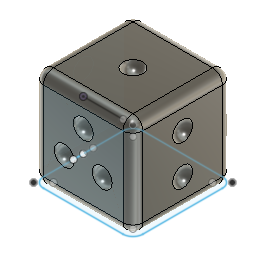
Radial D6 v1 (Autodesk Fusion 360 design; units mm, degrees)
Autodesk Fusion 360 part; units mm, degrees
note: some values were not read from the file. Chosen so that the rebuilt part matches the saved one: which face or edge a step refers to.
sketch "Sketch1" plane through (0, 0, 0) normal (0, 0, 1) x (1, 0, 0)
  line L0 (-20, 25) -> (20, 25)
  line L1 (25, 20) -> (25, -20)
  line L2 (20, -25) -> (-20, -25)
  line L3 (-25, -20) -> (-25, 20)
  arc A0 (-20, 25) -> (-25, 20) centre (-20, 20) ccw
  arc A1 (20, -25) -> (25, -20) centre (20, -20) ccw
  arc A2 (25, 20) -> (20, 25) centre (20, 20) ccw
  arc A3 (-25, -20) -> (-20, -25) centre (-20, -20) ccw
  point P0 (-25, 25)
  point P1 (25, 25)
  point P2 (-25, -25)
  dimension "d1" = 50
  dimension "d2" = 50
  dimension "d3" = 5
  dimension "d4" = 5
  dimension "d5" = 5
  dimension "d6" = 5
  constraint horizontal L0
  constraint vertical L1
  constraint horizontal L2
  constraint vertical L3
  constraint coincident P0 L0
  constraint coincident P0 L3
  constraint tangent L0 A0
  constraint tangent L3 A0
  constraint tangent L1 A1
  constraint tangent L2 A1
  constraint coincident P1 L0
  constraint coincident P1 L1
  constraint tangent L0 A2
  constraint tangent L1 A2
  constraint coincident P2 L2
  constraint coincident P2 L3
  constraint tangent L2 A3
  constraint tangent L3 A3
  measures "d1" distance of P0 P1
  measures "d2" distance of P0 P2
  measures "d3" radius of A0
  measures "d4" radius of A1
  measures "d5" radius of A2
  measures "d6" radius of A3
extrude "Extrude2" add sketch "Sketch1" along normal blind 50
fillet "Fillet3" radius 5 8 edges at (0, 25, 50) (-23.5355, 23.5355, 50) (-25, 0, 50) (-23.5355, -23.5355, 50) (0, -25, 50) (23.5355, -23.5355, 50) (25, 0, 50) (23.5355, 23.5355, 50)
fillet "Fillet4" radius 5 8 edges at (-23.5355, -23.5355, 0) (-25, 0, 0) (-23.5355, 23.5355, 0) (0, 25, 0) (23.5355, 23.5355, 0) (25, 0, 0) (23.5355, -23.5355, 0) (0, -25, 0)
sphere "SpherePrimitive1" cut diameter 10 placed x (-1, 0, 0) y (0, -1, 0) z (0, 0, 1) at (0, 0, 50)
sphere "SpherePrimitive2" cut diameter 10 placed x (1, 0, 0) y (0, 1, 0) z (0, 0, 1) at (13, 0, 0)
pattern_circular "C-Pattern1" count 6 over 360 about axis through (0, 0, 1.75) along (0, 0, 1) of 1 faces at (10.5214, -4.2931, 0.6526)
sphere "SpherePrimitive3" cut diameter 10 placed x (0, 1, 0) y (0, 0, 1) z (1, 0, 0) at (25, 0, 35)
sphere "SpherePrimitive4" cut diameter 10 placed x (0, 1, 0) y (0, 0, 1) z (1, 0, 0) at (25, 0, 15)
sphere "SpherePrimitive5" cut diameter 10 placed x (1, 0, 0) y (0, 0, 1) z (0, -1, 0) at (0, -25, 35)
move_face "MoveFace1" to x (1, 0, 0) y (0, 1, 0) z (0, 0, 1) at (0, 0, 1) 1 faces at (2.4786, -24.3474, 30.7069)
sketch "Sketch8" plane through (0, -25, 0) normal (0, -1, 0) x (1, 0, 0)
  circle A0 centre (0, 36) radius 5
  line L0 (-20, 5) -> (20, 5)
  line L1 (20, 5) -> (20, 45)
  line L2 (20, 45) -> (-20, 45)
  line L3 (-20, 45) -> (-20, 5)
  point P0 (0, 25)
sketch "Sketch9" plane through (0, 0, 0) normal (1, 0, 0) x (0, 1, 0)
  line L0 (-30, 25) -> (-20, 25)
  constraint horizontal L0
pattern_circular "C-Pattern2" count 3 over 360 about axis through (0, -30, 25) along (0, 1, 0) of 1 faces at (-2.4786, -24.3474, 31.7069)
sphere "SpherePrimitive6" cut diameter 10 placed x (-1, 0, 0) y (0, 0, 1) z (0, 1, 0) at (0, 25, 35)
move_face "MoveFace2" to x (1, 0, 0) y (0, 1, 0) z (0, 0, 1) at (0, 0, 2) 1 faces at (-2.4786, 24.3474, 30.7069)
pattern_circular "C-Pattern3" count 4 over 360 about axis through (0, -30, 25) along (0, 1, 0) of 1 faces at (2.4786, 24.3474, 32.7069)
sphere "SpherePrimitive7" cut diameter 10 placed x (0, -1, 0) y (0, 0, 1) z (-1, 0, 0) at (-25, 0, 37)
sketch "Sketch12" plane through (-25, 0, 0) normal (-1, 0, 0) x (0, -1, 0)
  circle A0 centre (0, 37) radius 5
  line L0 (-20, 5) -> (20, 5)
  line L1 (20, 5) -> (20, 45)
  line L2 (20, 45) -> (-20, 45)
  line L3 (-20, 45) -> (-20, 5)
  point P0 (0, 25)
sketch "Sketch14" plane through (0, 0, 0) normal (0, 1, 0) x (1, 0, 0)
  line L0 (-25, -25) -> (-5, -25)
  point P0 (-25, -25)
  constraint coincident P0 L0.start
  constraint horizontal L0
pattern_circular "C-Pattern4" count 5 over 360 about axis through (-25, 0, 25) along (1, 0, 0) of 1 faces at (-24.3474, 2.4786, 32.7069)
